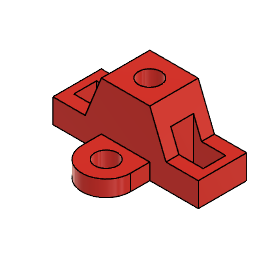
MARS_1_ME25B1021 (Autodesk Fusion 360 design; units mm, degrees)
part number: 2026-05-31-12-03-16-631
Autodesk Fusion 360 part; units mm, degrees
sketch "Sketch1" plane through (0, 0, 0) normal (0, 0, 1) x (1, 0, 0)
  line L0 (0, 0) -> (90, 0)
  line L1 (90, 0) -> (90, 30)
  line L2 (90, 30) -> (0, 30)
  line L3 (0, 30) -> (0, 0)
  dimension "d2" = 90
  dimension "d3" = 30
  constraint horizontal L0
  constraint vertical L1
  constraint horizontal L2
  constraint vertical L3
  constraint coincident L0.start L3.end
  measures "d2" distance of L0.start L0.end
  measures "d3" distance of L0.start L2.end
extrude "Extrude1" add sketch "Sketch1" along normal blind 40
sketch "Sketch2" plane through (0, 0, 0) normal (0, -1, 0) x (1, 0, 0)
  line L0 (0, 0) -> (90, 0)
  line L1 (90, 0) -> (90, 40)
  line L2 (90, 40) -> (0, 40)
  line L3 (0, 40) -> (0, 0)
  line L4 (30, 40) -> (20, 15)
  line L5 (20, 15) -> (0, 15)
  line L6 (30, 40) -> (0, 40)
  line L7 (0, 15) -> (0, 40)
  line L8 (45, 40) -> (45, 0) construction
  line L9 (60, 40) -> (70, 15)
  line L10 (60, 40) -> (90, 40)
  line L11 (90, 15) -> (90, 40)
  line L12 (70, 15) -> (90, 15)
  dimension "d8" = 15
  dimension "d11" = 30
  dimension "d12" = 50
  constraint coincident L2 L4.start
  constraint coincident L3 L5.end
  constraint perpendicular L3 L5
  constraint coincident L2.end L3.start
  constraint midpoint L2 L8.start
  constraint midpoint L0 L8.end
  constraint symmetric L4.start L8 L9.start
  constraint symmetric L4.end L8 L9.end
  constraint symmetric L5.end L8 L11.start
  constraint symmetric L2.end L8 L1.end
  measures "d8" distance of L0.start L5.end
  measures "d11" distance of L4.start L9.start
  measures "d12" distance of L4.end L9.end
extrude "Extrude2" cut sketch "Sketch2" against normal blind 55 contours L2 L3 L4 L5 L6 L7 | L1 L2 L9 L10 L11 L12
sketch "Sketch3" plane through (0, 0, 40) normal (0, 0, 1) x (-1, 0, 0)
  line L0 (-30, -30) -> (-30, 0)
  line L1 (-30, 0) -> (-60, 0)
  line L2 (-60, 0) -> (-60, -30)
  line L3 (-60, -30) -> (-30, -30)
  line L4 (-45, -30) -> (-45, 0) construction
  circle A0 centre (-45, -15) radius 7 construction
  line L5 (-5, -22) -> (-25, -22)
  line L6 (-25, -22) -> (-25, -8)
  line L7 (-25, -8) -> (-5, -8)
  line L8 (-5, -8) -> (-5, -22)
  line L9 (-20, 0) -> (0, 0)
  line L10 (0, -30) -> (-20, -30)
  line L11 (0, 0) -> (0, -30)
  line L12 (-65, -8) -> (-85, -8)
  line L13 (-85, -22) -> (-65, -22)
  line L14 (-85, -8) -> (-85, -22)
  line L15 (-65, -22) -> (-65, -8)
  circle A1 centre (-45, -15) radius 7
  dimension "d15" = 14
  dimension "d16" = 20
  dimension "d17" = 14
  dimension "d18" = 8
  dimension "d20" = 5
  dimension "d21" = 14
  constraint midpoint L3 L4.start
  constraint midpoint L1 L4.end
  constraint midpoint L4 A0.centre
  constraint horizontal L5
  constraint vertical L6
  constraint horizontal L7
  constraint vertical L8
  constraint symmetric L4 L5.start L13.start
  constraint symmetric L4 L5.end L13.end
  constraint symmetric L4 L6.end L12.start
  constraint symmetric L4 L7.end L12.end
  constraint concentric A0 A1
  measures "d15" diameter of A0
  measures "d16" distance of L5.start L5.end
  measures "d17" distance of L5.start L7.end
  measures "d18" distance of L7.end L9
  measures "d20" distance of L7.end L11
  measures "d21" diameter of A1
extrude "Extrude3" cut sketch "Sketch3" against normal through all contours L5 L6 L7 L8 | L12 L13 L14 L15 | A1
sketch "Sketch4" plane through (0, 0, 0) normal (0, 0, 1) x (1, 0, 0)
  line L0 (30, 0) -> (60, 0)
  line L1 (60, 0) -> (60, -10)
  line L2 (60, -10) -> (60, -12)
  arc A0 (30, -12) -> (60, -12) centre (45, -12) ccw
  line L3 (30, -12) -> (30, 0)
  circle A1 centre (45, -12) radius 7
  point P0 (30, 0)
  dimension "d23" = 15
  dimension "d24" = 30
  dimension "d25" = 14
  dimension "d26" = 12
  constraint horizontal L0
  constraint perpendicular L0 L1
  constraint perpendicular L0 L2
  constraint tangent L2 A0
  constraint perpendicular L0 L3
  constraint coincident P0 L0.start
  constraint concentric A0 A1
  measures "d23" radius of A0
  measures "d24" distance of P0 L0.end
  measures "d25" diameter of A1
  measures "d26" distance of L0 A0.centre
extrude "Extrude4" add sketch "Sketch4" along normal blind 10
